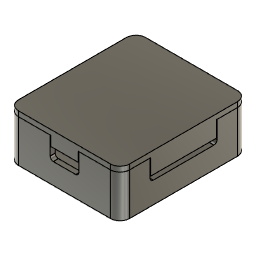
usbwledc-case (Autodesk Fusion 360 design; units mm, degrees)
Autodesk Fusion 360 part; units mm, degrees
sketch "Skizze1" plane through (0, 0, 0) normal (0, 0, 1) x (1, 0, 0)
  line L0 (0, 0) -> (34.8, 0)
  line L1 (34.8, 0) -> (34.8, 39.8)
  line L2 (34.8, 39.8) -> (0, 39.8)
  line L3 (0, 39.8) -> (0, 0)
  line L4 (33.2, 1.6) -> (1.6, 1.6)
  line L5 (1.6, 1.6) -> (1.6, 38.2)
  line L6 (1.6, 38.2) -> (33.2, 38.2)
  line L7 (33.2, 38.2) -> (33.2, 1.6)
  line L8 (33.2, 1.6) -> (1.6, 38.2) construction
  line L9 (1.6, 1.6) -> (33.2, 38.2) construction
  line L10 (33.2, 1.6) -> (29.4, 1.6) construction
  line L11 (29.4, 1.6) -> (29.4, 5.4) construction
  line L12 (1.6, 1.6) -> (5.4, 1.6) construction
  line L13 (5.4, 1.6) -> (5.4, 5.4) construction
  circle A0 centre (29.4, 5.4) radius 1.4
  circle A1 centre (5.4, 5.4) radius 1.4
  line L14 (5.4, 1.6) -> (7.9, 1.6) construction
  line L15 (7.9, 1.6) -> (7.9, 5.4)
  arc A2 (7.9, 5.4) -> (5.4, 7.9) centre (5.4, 5.4) ccw
  line L16 (5.4, 7.9) -> (1.6, 7.9)
  line L17 (29.4, 1.6) -> (26.9, 1.6) construction
  line L18 (33.2, 38.2) -> (29.4, 38.2) construction
  line L19 (1.6, 38.2) -> (5.4, 38.2) construction
  line L20 (5.4, 38.2) -> (5.4, 34.4) construction
  line L21 (29.4, 38.2) -> (29.4, 34.4) construction
  circle A3 centre (29.4, 34.4) radius 1.4
  circle A4 centre (5.4, 34.4) radius 1.4
  line L22 (29.4, 38.2) -> (26.9, 38.2) construction
  line L23 (5.4, 38.2) -> (7.9, 38.2) construction
  line L24 (26.9, 38.2) -> (26.9, 34.4)
  line L25 (7.9, 38.2) -> (7.9, 34.4)
  arc A5 (5.4, 31.9) -> (7.9, 34.4) centre (5.4, 34.4) ccw
  arc A6 (26.9, 34.4) -> (29.4, 31.9) centre (29.4, 34.4) ccw
  line L26 (5.4, 31.9) -> (1.6, 31.9)
  line L27 (29.4, 31.9) -> (33.2, 31.9)
  line L28 (26.9, 1.6) -> (26.9, 5.4)
  arc A7 (29.4, 7.9) -> (26.9, 5.4) centre (29.4, 5.4) ccw
  line L29 (29.4, 7.9) -> (33.2, 7.9)
  point P0 (17.4, 19.9)
  dimension "d15" = 34.8
  dimension "d16" = 39.8
  dimension "d17" = 31.6
  dimension "d18" = 36.6
  dimension "d19" = 3.8
  dimension "d20" = 3.8
  dimension "d21" = 3.8
  dimension "d22" = 3.8
  dimension "d23" = 2.8
  dimension "d24" = 2.8
  dimension "d27" = 2.5
  dimension "d28" = 3.8
  dimension "d29" = 2.5
  dimension "d30" = 3.8
  dimension "d31" = 3.8
  dimension "d32" = 3.8
  dimension "d33" = 3.8
  dimension "d34" = 2.8
  dimension "d35" = 2.8
  dimension "d36" = 2.5
  dimension "d37" = 2.5
  dimension "d38" = 3.8
  dimension "d39" = 3.8
  dimension "d40" = 3.8
  constraint horizontal L0
  constraint vertical L1
  constraint horizontal L2
  constraint vertical L3
  constraint coincident L0.start L3.end
  constraint horizontal L4
  constraint perpendicular L4 L5
  constraint parallel L4 L6
  constraint parallel L5 L7
  constraint coincident L8 P0
  constraint coincident L9 P0
  constraint perpendicular L7 L10
  constraint perpendicular L4 L11
  constraint perpendicular L5 L12
  constraint perpendicular L4 L13
  constraint coincident L11.end A0.centre
  constraint coincident L13.end A1.centre
  constraint perpendicular L13 L14
  constraint perpendicular L14 L15
  constraint coincident L5 L16.end
  constraint tangent A2 L16
  constraint perpendicular L5 L16
  constraint perpendicular L11 L17
  constraint perpendicular L7 L18
  constraint perpendicular L5 L19
  constraint perpendicular L19 L20
  constraint perpendicular L6 L21
  constraint coincident L21.end A3.centre
  constraint coincident L20.end A4.centre
  constraint perpendicular L21 L22
  constraint perpendicular L21 L23
  constraint perpendicular L22 L24
  constraint perpendicular L23 L25
  constraint coincident L5 L26.end
  constraint tangent A5 L26
  constraint perpendicular L5 L26
  constraint coincident L7 L27.end
  constraint tangent A6 L27
  constraint perpendicular L7 L27
  constraint perpendicular L17 L28
  constraint coincident L7 L29.end
  constraint tangent A7 L29
  constraint perpendicular L7 L29
  measures "d15" distance of L0.start L0.end
  measures "d16" distance of L0.start L2.end
  measures "d17" distance of L5.end L6.end
  measures "d18" distance of L4.end L5.end
  measures "d19" distance of L4.start L10.end
  measures "d20" distance of L10.end L11.end
  measures "d21" distance of L4.end L12.end
  measures "d22" distance of L12.end L13.end
  measures "d23" diameter of A0
  measures "d24" diameter of A1
  measures "d27" distance of L12.end L14.end
  measures "d28" distance of L14.end L15.end
  measures "d29" distance of L10.end L17.end
  measures "d30" distance of L6.end L18.end
  measures "d31" distance of L5.end L19.end
  measures "d32" distance of L19.end L20.end
  measures "d33" distance of L18.end L21.end
  measures "d34" diameter of A3
  measures "d35" diameter of A4
  measures "d36" distance of L18.end L22.end
  measures "d37" distance of L19.end L23.end
  measures "d38" distance of L22.end L24.end
  measures "d39" distance of L23.end L25.end
  measures "d40" distance of L17.end L28.end
extrude "Extrusion1" add sketch "Skizze1" along normal blind 1.6 contours L4 L5 L6 L7 L15 A2 L16 L24 L25 A5 A6 L26 L27 L28 A7 L29 makes body 1
extrude "Extrusion2" add sketch "Skizze1" along normal blind 5.1 contours L4 L7 L28 A7 L29 | L4 L5 L15 A2 L16 | L6 L7 L24 A6 L27 | L5 L6 L25 A5 L26 bodies 1
extrude "Extrusion3" add sketch "Skizze1" along normal blind 13.2 contours L0 L1 L2 L3 bodies 1
extrude "Extrusion4" add sketch "Skizze1" along normal blind 6.7 contours A0 | A1 | A3 | A4 bodies 1
sketch "Skizze2" plane through (0, 0, 1.6) normal (0, 0, 1) x (-1, 0, 0)
  line L0 (-26.9, -1.6) -> (-26.9, -5.4)
  arc A0 (-29.4, -7.9) -> (-26.9, -5.4) centre (-29.4, -5.4) ccw
  line L1 (-29.4, -7.9) -> (-33.2, -7.9)
  line L2 (-33.2, -7.9) -> (-33.2, -31.9)
  line L3 (-33.2, -31.9) -> (-29.4, -31.9)
  arc A1 (-26.9, -34.4) -> (-29.4, -31.9) centre (-29.4, -34.4) ccw
  line L4 (-26.9, -34.4) -> (-26.9, -38.2)
  line L5 (-26.9, -38.2) -> (-7.9, -38.2)
  line L6 (-7.9, -38.2) -> (-7.9, -34.4)
  arc A2 (-5.4, -31.9) -> (-7.9, -34.4) centre (-5.4, -34.4) ccw
  line L7 (-5.4, -31.9) -> (-1.6, -31.9)
  line L8 (-1.6, -31.9) -> (-1.6, -7.9)
  line L9 (-1.6, -7.9) -> (-5.4, -7.9)
  arc A3 (-7.9, -5.4) -> (-5.4, -7.9) centre (-5.4, -5.4) ccw
  line L10 (-7.9, -5.4) -> (-7.9, -1.6)
  line L11 (-7.9, -1.6) -> (-26.9, -1.6)
  line L12 (-33.2, -7.9) -> (-32.6, -7.9)
  line L13 (-32.6, -7.9) -> (-32.6, -31.9)
  line L14 (-32.6, -31.9) -> (-33.2, -31.9)
  line L15 (-33.2, -31.9) -> (-33.2, -7.9)
  dimension "d49" = 0.6
  constraint coincident L1.end L2.start
  constraint coincident L1 L12.end
  constraint coincident L3 L13.end
  constraint perpendicular L3 L13
  constraint coincident L2.end L3.start
  measures "d49" distance of L1.end L12.end
extrude "Extrusion5" add sketch "Skizze2" along normal blind 5.1 contours L1 L2 L3 L12 L13 L14 L15 bodies 1
sketch "Skizze3" plane through (0, 0, 0) normal (0, -1, 0) x (1, 0, 0)
  line L0 (0, 0) -> (34.8, 0)
  line L1 (34.8, 0) -> (34.8, 13.2)
  line L2 (34.8, 13.2) -> (0, 13.2)
  line L3 (0, 13.2) -> (0, 0)
  line L4 (17.4, 0) -> (17.4, 6.5) construction
  line L5 (17.4, 6.5) -> (21.9, 6.5)
  line L6 (17.4, 6.5) -> (12.9, 6.5)
  line L7 (12.9, 6.5) -> (12.9, 13.2)
  line L8 (21.9, 6.5) -> (21.9, 13.2)
  line L9 (21.9, 13.2) -> (12.9, 13.2)
  dimension "d52" = 6.5
  dimension "d55" = 4.5
  dimension "d56" = 4.5
  constraint midpoint L0 L4.start
  constraint perpendicular L0 L4
  constraint perpendicular L4 L5
  constraint perpendicular L4 L6
  constraint coincident L2 L7.end
  constraint perpendicular L2 L7
  constraint coincident L2 L8.end
  constraint perpendicular L2 L8
  measures "d52" distance of L4.start L4.end
  measures "d55" distance of L4.end L5.end
  measures "d56" distance of L4.end L6.end
extrude "Extrusion6" cut sketch "Skizze3" against normal blind 1.6 contours L2 L5 L6 L7 L8 L9 bodies 1
sketch "Skizze4" plane through (34.8, 0, 0) normal (1, 0, 0) x (0, 1, 0)
  line L0 (0, 0) -> (39.8, 0)
  line L1 (39.8, 0) -> (39.8, 13.2)
  line L2 (39.8, 13.2) -> (0, 13.2)
  line L3 (0, 13.2) -> (0, 0)
  line L4 (19.9, 0) -> (19.9, 6.7) construction
  line L5 (19.9, 6.7) -> (30.4, 6.7)
  line L6 (19.9, 6.7) -> (9.4, 6.7)
  line L7 (9.4, 6.7) -> (9.4, 13.2)
  line L8 (30.4, 6.7) -> (30.4, 13.2)
  line L9 (30.4, 13.2) -> (9.4, 13.2)
  dimension "d59" = 6.7
  dimension "d60" = 10.5
  dimension "d61" = 10.5
  constraint midpoint L0 L4.start
  constraint perpendicular L0 L4
  constraint perpendicular L1 L5
  constraint perpendicular L4 L6
  constraint coincident L2 L7.end
  constraint perpendicular L2 L7
  constraint coincident L2 L8.end
  constraint perpendicular L2 L8
  measures "d59" distance of L4.start L4.end
  measures "d60" distance of L4.end L5.end
  measures "d61" distance of L4.end L6.end
extrude "Extrusion7" cut sketch "Skizze4" against normal blind 1.6 contours L2 L5 L6 L7 L8 L9 bodies 1
ref_plane "Arbeitsebene1" through (0, 0, 13.2) normal (0, 0, 1) x (1, 0, 0)
ref_plane "Arbeitsebene2" through (0, 19.9, 0) normal (0, 1, 0) x (0, 0, 1)
sketch "Skizze6" plane through (0, 0, 13.2) normal (0, 0, 1) x (1, 0, 0)
  line L0 (2, 2) -> (2, 37.8)
  line L1 (5.4, 2) -> (5.4, 5.4) construction
  line L2 (32.8, 37.8) -> (32.8, 2)
  line L3 (29.4, 2) -> (26.9, 2) construction
  line L4 (29.4, 7.9) -> (32.8, 7.9)
  line L5 (32.8, 37.8) -> (29.4, 37.8) construction
  line L6 (5.4, 2) -> (7.9, 2) construction
  line L7 (32.8, 2) -> (29.4, 2) construction
  line L8 (34.8, 0) -> (34.8, 39.8)
  line L9 (2, 37.8) -> (5.4, 37.8) construction
  line L10 (5.4, 37.8) -> (7.9, 37.8) construction
  arc A0 (29.4, 7.9) -> (26.9, 5.4) centre (29.4, 5.4) ccw
  line L11 (29.4, 2) -> (29.4, 5.4) construction
  line L12 (0, 39.8) -> (0, 0)
  line L13 (26.9, 2) -> (26.9, 5.4)
  line L14 (2, 2) -> (5.4, 2) construction
  line L15 (2, 2) -> (32.8, 37.8) construction
  line L16 (2, 37.8) -> (32.8, 37.8)
  line L17 (34.8, 39.8) -> (0, 39.8)
  line L18 (0, 0) -> (34.8, 0)
  line L19 (32.8, 2) -> (2, 37.8) construction
  line L20 (32.8, 2) -> (2, 2)
  line L21 (29.4, 37.8) -> (26.9, 37.8) construction
  line L22 (7.9, 2) -> (7.9, 5.4)
  arc A1 (7.9, 5.4) -> (5.4, 7.9) centre (5.4, 5.4) ccw
  line L23 (5.4, 5.4) -> (7.9, 5.4) construction
  line L24 (5.4, 5.4) -> (5.4, 7.9) construction
  line L25 (5.4, 7.9) -> (2, 7.9)
  line L26 (7.9, 37.8) -> (7.9, 34.4)
  line L27 (26.9, 37.8) -> (26.9, 34.4)
  line L28 (29.4, 37.8) -> (29.4, 34.4) construction
  line L29 (5.4, 37.8) -> (5.4, 34.4) construction
  arc A2 (5.4, 31.9) -> (7.9, 34.4) centre (5.4, 34.4) ccw
  line L30 (5.4, 34.4) -> (5.4, 31.9) construction
  line L31 (5.4, 34.4) -> (7.9, 34.4) construction
  arc A3 (26.9, 34.4) -> (29.4, 31.9) centre (29.4, 34.4) ccw
  line L32 (29.4, 34.4) -> (26.9, 34.4) construction
  line L33 (29.4, 34.4) -> (29.4, 31.9) construction
  line L34 (5.4, 31.9) -> (2, 31.9)
  line L35 (29.4, 31.9) -> (32.8, 31.9)
  point P0 (17.4, 19.9)
  dimension "d89" = 34.8
  dimension "d90" = 39.8
  dimension "d91" = 30.8
  dimension "d92" = 35.8
  dimension "d93" = 3.4
  dimension "d94" = 3.4
  dimension "d95" = 3.4
  dimension "d96" = 3.4
  dimension "d99" = 2.5
  dimension "d101" = 2.5
  dimension "d102" = 3.4
  dimension "d103" = 3.4
  dimension "d108" = 2.5
  dimension "d109" = 2.5
  dimension "d112" = 3.4
  dimension "d118" = 3.4
  dimension "d119" = 90
  dimension "d120" = 3.4
  dimension "d121" = 3.4
  dimension "d122" = 3.4
  dimension "d123" = 3.4
  dimension "d124" = 90
  dimension "d125" = 90
  constraint horizontal L18
  constraint vertical L8
  constraint horizontal L17
  constraint vertical L12
  constraint coincident L12.end L18.start
  constraint horizontal L20
  constraint perpendicular L0 L20
  constraint parallel L16 L20
  constraint parallel L0 L2
  constraint coincident P0 L19
  constraint coincident P0 L15
  constraint perpendicular L2 L7
  constraint perpendicular L11 L20
  constraint perpendicular L0 L14
  constraint perpendicular L1 L20
  constraint perpendicular L1 L6
  constraint perpendicular L3 L11
  constraint perpendicular L2 L5
  constraint perpendicular L0 L9
  constraint perpendicular L3 L13
  constraint coincident L4.end L2
  constraint tangent L4 A0
  constraint perpendicular L2 L4
  constraint perpendicular L20 L22
  constraint coincident L0 L25.end
  constraint tangent A1 L25
  constraint perpendicular L10 L26
  constraint perpendicular L21 L27
  constraint perpendicular L5 L28
  constraint perpendicular L10 L29
  constraint coincident L29.end A2.centre
  constraint coincident L28.end A3.centre
  constraint coincident L0 L34.end
  constraint tangent A2 L34
  constraint perpendicular L0 L34
  constraint coincident L2 L35.end
  constraint tangent A3 L35
  constraint perpendicular L2 L35
  measures "d89" distance of L8.start L12.end
  measures "d90" distance of L12.end L12.start
  measures "d91" distance of L2.start L0.end
  measures "d92" distance of L0.start L0.end
  measures "d93" distance of L2.end L3.start
  measures "d94" distance of L3.start A0.centre
  measures "d95" distance of L0.start L1.start
  measures "d96" distance of L1.start L1.end
  measures "d99" distance of L1.start L6.end
  measures "d101" distance of L3.end L3.start
  measures "d102" distance of L2.start L5.end
  measures "d103" distance of L0.end L9.end
  measures "d108" distance of L21.end L5.end
  measures "d109" distance of L10.end L9.end
  measures "d112" distance of L3.end A0.end
  measures "d118" distance of L6.end L22.end
  measures "d119" angle of L23 L24
  measures "d120" distance of L10.end L26.end
  measures "d121" distance of L21.end L27.end
  measures "d122" distance of L5.end L28.end
  measures "d123" distance of L9.end L29.end
  measures "d124" angle of L30 L31
  measures "d125" angle of L32 L33
extrude "Extrusion8" add sketch "Skizze6" along normal blind 1.6 separate body contours L0 L20 L22 A1 L25 | L0 L2 L4 A0 L13 L16 L20 L22 A1 L25 L26 L27 A2 A3 L34 L35 | L0 L16 L26 A2 L34 | L2 L4 A0 L13 L20 | L2 L16 L27 A3 L35 | L8 L12 L17 L18 makes body 2
extrude "Extrusion9" add sketch "Skizze6" against normal blind 6.4 contours L0 L20 L22 A1 L25 | L0 L16 L26 A2 L34 | L2 L4 A0 L13 L20 | L2 L16 L27 A3 L35 bodies 2
ref_plane "Arbeitsebene3" through (0, 0, 6.7) normal (0, 0, 1) x (1, 0, 0)
sketch "Skizze7" plane through (0, 0, 13.2) normal (0, 0, -1) x (1, 0, 0)
  line L0 (32.8, -37.8) -> (26.9, -37.8)
  line L1 (26.9, -37.8) -> (26.9, -34.4)
  arc A0 (29.4, -31.9) -> (26.9, -34.4) centre (29.4, -34.4) ccw
  line L2 (29.4, -31.9) -> (32.8, -31.9)
  line L3 (32.8, -31.9) -> (32.8, -37.8)
  line L4 (2, -2) -> (7.9, -2)
  line L5 (7.9, -2) -> (7.9, -5.4)
  arc A1 (5.4, -7.9) -> (7.9, -5.4) centre (5.4, -5.4) ccw
  line L6 (5.4, -7.9) -> (2, -7.9)
  line L7 (2, -7.9) -> (2, -2)
  line L8 (26.9, -5.4) -> (26.9, -2)
  line L9 (26.9, -2) -> (32.8, -2)
  line L10 (32.8, -2) -> (32.8, -7.9)
  line L11 (32.8, -7.9) -> (29.4, -7.9)
  arc A2 (26.9, -5.4) -> (29.4, -7.9) centre (29.4, -5.4) ccw
  line L12 (7.9, -34.4) -> (7.9, -37.8)
  line L13 (7.9, -37.8) -> (2, -37.8)
  line L14 (2, -37.8) -> (2, -31.9)
  line L15 (2, -31.9) -> (5.4, -31.9)
  arc A3 (7.9, -34.4) -> (5.4, -31.9) centre (5.4, -34.4) ccw
  line L16 (34.8, 0) -> (0, 0)
  line L17 (0, 0) -> (0, -39.8)
  line L18 (0, -39.8) -> (34.8, -39.8)
  line L19 (34.8, -39.8) -> (34.8, 0)
  line L20 (17.4, 0) -> (21.7, 0)
  line L21 (21.7, 0) -> (21.7, -1.6)
  line L22 (21.7, -1.6) -> (13.1, -1.6)
  line L23 (13.1, -1.6) -> (13.1, 0)
  line L24 (13.1, 0) -> (17.4, 0)
  dimension "d127" = 4.3
  dimension "d128" = 1.6
  dimension "d129" = 8.6
  constraint midpoint L16 L20.start
  constraint coincident L16 L20.end
  constraint perpendicular L20 L21
  constraint perpendicular L21 L22
  constraint coincident L16 L23.end
  constraint perpendicular L16 L23
  measures "d127" distance of L20.start L20.end
  measures "d128" distance of L20.end L21.end
  measures "d129" distance of L21.end L22.end
extrude "Extrusion10" add sketch "Skizze7" along normal blind 3 contours L16 L20 L21 L22 L23 L24 bodies 2
sketch "Skizze8" plane through (0, 0, 13.2) normal (0, 0, -1) x (1, 0, 0)
  line L0 (21.7, 0) -> (21.7, -1.6)
  line L1 (21.7, -1.6) -> (13.1, -1.6)
  line L2 (13.1, -1.6) -> (13.1, 0)
  line L3 (13.1, 0) -> (0, 0)
  line L4 (0, 0) -> (0, -39.8)
  line L5 (0, -39.8) -> (34.8, -39.8)
  line L6 (34.8, -39.8) -> (34.8, 0)
  line L7 (34.8, 0) -> (21.7, 0)
  line L8 (7.9, -34.4) -> (7.9, -37.8)
  line L9 (7.9, -37.8) -> (2, -37.8)
  line L10 (2, -37.8) -> (2, -31.9)
  line L11 (2, -31.9) -> (5.4, -31.9)
  arc A0 (7.9, -34.4) -> (5.4, -31.9) centre (5.4, -34.4) ccw
  line L12 (26.9, -5.4) -> (26.9, -2)
  line L13 (26.9, -2) -> (32.8, -2)
  line L14 (32.8, -2) -> (32.8, -7.9)
  line L15 (32.8, -7.9) -> (29.4, -7.9)
  arc A1 (26.9, -5.4) -> (29.4, -7.9) centre (29.4, -5.4) ccw
  line L16 (2, -2) -> (7.9, -2)
  line L17 (7.9, -2) -> (7.9, -5.4)
  arc A2 (5.4, -7.9) -> (7.9, -5.4) centre (5.4, -5.4) ccw
  line L18 (5.4, -7.9) -> (2, -7.9)
  line L19 (2, -7.9) -> (2, -2)
  line L20 (32.8, -37.8) -> (26.9, -37.8)
  line L21 (26.9, -37.8) -> (26.9, -34.4)
  arc A3 (29.4, -31.9) -> (26.9, -34.4) centre (29.4, -34.4) ccw
  line L22 (29.4, -31.9) -> (32.8, -31.9)
  line L23 (32.8, -31.9) -> (32.8, -37.8)
  line L24 (34.8, -19.9) -> (34.8, -30.2)
  line L25 (34.8, -30.2) -> (32.6, -30.2)
  line L26 (32.6, -30.2) -> (32.6, -9.6)
  line L27 (32.6, -9.6) -> (34.8, -9.6)
  line L28 (34.8, -9.6) -> (34.8, -19.9)
  dimension "d132" = 10.3
  dimension "d133" = 2.2
  dimension "d134" = 20.6
  constraint midpoint L6 L24.start
  constraint parallel L6 L24
  constraint perpendicular L24 L25
  constraint perpendicular L25 L26
  constraint coincident L6 L27.end
  constraint perpendicular L6 L27
  measures "d132" distance of L24.start L24.end
  measures "d133" distance of L24.end L25.end
  measures "d134" distance of L25.end L26.end
extrude "Extrusion11" add sketch "Skizze8" along normal blind 5 contours L6 L24 L25 L26 L27 L28 bodies 2
sketch "Skizze9" plane through (32.8, 0, 0) normal (1, 0, 0) x (0, 1, 0)
  line L0 (7.9, 13.2) -> (2, 13.2)
  line L1 (2, 13.2) -> (2, 6.8)
  line L2 (2, 6.8) -> (7.9, 6.8)
  line L3 (7.9, 6.8) -> (7.9, 13.2)
  line L4 (2, 13.2) -> (7.9, 6.8) construction
  line L5 (2, 6.8) -> (7.9, 13.2) construction
  constraint coincident L0.end L1.start
  constraint coincident L2.end L3.start
  constraint coincident L1.end L2.start
  constraint coincident L0.start L3.end
sketch "Skizze10" plane through (32.8, 0, 0) normal (1, 0, 0) x (0, 1, 0)
  line L0 (37.8, 13.2) -> (31.9, 13.2)
  line L1 (31.9, 13.2) -> (31.9, 6.8)
  line L2 (31.9, 6.8) -> (37.8, 6.8)
  line L3 (37.8, 6.8) -> (37.8, 13.2)
  line L4 (31.9, 13.2) -> (37.8, 6.8) construction
  line L5 (31.9, 6.8) -> (37.8, 13.2) construction
  constraint coincident L0.end L1.start
  constraint coincident L2.end L3.start
  constraint coincident L1.end L2.start
  constraint coincident L0.start L3.end
sketch "Skizze11" plane through (2, 0, 0) normal (-1, 0, 0) x (0, -1, 0)
  line L0 (-31.9, 13.2) -> (-37.8, 13.2)
  line L1 (-37.8, 13.2) -> (-37.8, 6.8)
  line L2 (-37.8, 6.8) -> (-31.9, 6.8)
  line L3 (-31.9, 6.8) -> (-31.9, 13.2)
  line L4 (-37.8, 6.8) -> (-31.9, 13.2) construction
  line L5 (-37.8, 13.2) -> (-31.9, 6.8) construction
  constraint coincident L1.end L2.start
  constraint coincident L0.start L3.end
  constraint coincident L0.end L1.start
  constraint coincident L2.end L3.start
sketch "Skizze12" plane through (2, 0, 0) normal (-1, 0, 0) x (0, -1, 0)
  line L0 (-2, 13.2) -> (-7.9, 13.2)
  line L1 (-7.9, 13.2) -> (-7.9, 6.8)
  line L2 (-7.9, 6.8) -> (-2, 6.8)
  line L3 (-2, 6.8) -> (-2, 13.2)
  line L4 (-7.9, 13.2) -> (-2, 6.8) construction
  line L5 (-7.9, 6.8) -> (-2, 13.2) construction
  constraint coincident L0.end L1.start
  constraint coincident L2.end L3.start
  constraint coincident L1.end L2.start
  constraint coincident L0.start L3.end
sphere "Grundkörper Kugel1" add diameter 2.4 placed x (0, -1, 0) y (0, 0, 1) z (-1, 0, 0) at (2, 4.95, 10) bodies 2
sphere "Grundkörper Kugel2" add diameter 2.4 placed x (0, -1, 0) y (0, 0, 1) z (-1, 0, 0) at (2, 34.85, 10) bodies 2
sphere "Grundkörper Kugel3" add diameter 2.4 placed x (0, 1, 0) y (0, 0, 1) z (1, 0, 0) at (32.8, 4.95, 10) bodies 2
sphere "Grundkörper Kugel4" add diameter 2.4 placed x (0, 1, 0) y (0, 0, 1) z (1, 0, 0) at (32.8, 34.85, 10) bodies 2
sphere "Grundkörper Kugel5" cut diameter 2.5 placed x (0, -1, 0) y (0, 0, 1) z (-1, 0, 0) at (2, 4.95, 10) bodies 1
sphere "Grundkörper Kugel6" cut diameter 2.5 placed x (0, -1, 0) y (0, 0, 1) z (-1, 0, 0) at (2, 34.85, 10) bodies 1
sphere "Grundkörper Kugel7" cut diameter 2.5 placed x (0, 1, 0) y (0, 0, 1) z (1, 0, 0) at (32.8, 4.95, 10) bodies 1
sphere "Grundkörper Kugel8" cut diameter 2.5 placed x (0, 1, 0) y (0, 0, 1) z (1, 0, 0) at (32.8, 34.85, 10) bodies 1
fillet "Abrundung1" radius 1.5 8 edges at (33.2, 1.6, 9.15) (33.2, 38.2, 9.15) (1.6, 38.2, 9.15) (1.6, 1.6, 9.15) (32.8, 37.8, 10) (32.8, 2, 10) (2, 37.8, 10) (2, 2, 10) on bodies 1 2
fillet "Abrundung2" radius 3 8 edges at (0, 39.8, 6.6) (34.8, 39.8, 6.6) (0, 0, 6.6) (34.8, 0, 6.6) (0, 39.8, 14) (34.8, 39.8, 14) (0, 0, 14) (34.8, 0, 14) on bodies 1 2
fillet "Abrundung3" radius 2.5 1 edges at (32.6, 19.9, 13.2) on bodies 2
fillet "Abrundung4" radius 1 2 edges at (21.9, 0.8, 6.5) (12.9, 0.8, 6.5) on bodies 1
fillet "Abrundung5" radius 1 2 edges at (34, 30.4, 6.7) (34, 9.4, 6.7) on bodies 1
equation "platineBreite = 30 mm"
equation "platineLänge = 35 mm"
equation "platineAbstandUnten = 3.5 mm"
equation "platineAbstandOben = 6.5 mm"
equation "platineLochAbstand = 3 mm"
equation "platineLochDurchmesser = 3.2 mm"
equation "platineDicke = 1.6 mm"
equation "wandstärke = 1.6 mm"
equation "platineAbstandBreite = 0.8 mm"
equation "platineAbstandLänge = platineAbstandBreite"
equation "platinePadsLänge = 21 mm"
equation "platineKabelDicke = 1.5 mm"
equation "toleranz = 0.2 mm"
equation "d15 = platineBreite + ( ( wandstärke + platineAbstandBreite ) * 2 )"
equation "d16 = platineLänge + ( ( platineAbstandLänge + wandstärke ) * 2 )"
equation "d17 = platineBreite + ( platineAbstandBreite * 2 )"
equation "d18 = platineLänge + ( platineAbstandLänge * 2 )"
equation "d19 = platineLochAbstand + platineAbstandBreite"
equation "d20 = platineAbstandLänge + platineLochAbstand"
equation "d21 = platineLochAbstand + platineAbstandBreite"
equation "d22 = platineLochAbstand + platineAbstandLänge"
equation "d23 = platineLochDurchmesser - ( toleranz * 2 )"
equation "d24 = platineLochDurchmesser - ( toleranz * 2 )"
equation "platineLochRing = 5 mm"
equation "d27 = platineLochRing / 2"
equation "d28 = platineLochAbstand + platineAbstandLänge"
equation "d29 = platineLochRing / 2"
equation "d30 = platineLochAbstand + platineAbstandBreite"
equation "d31 = platineLochAbstand + platineAbstandBreite"
equation "d32 = platineLochAbstand + platineAbstandLänge"
equation "d33 = platineLochAbstand + platineAbstandLänge"
equation "d34 = platineLochDurchmesser - ( 2 * toleranz )"
equation "d35 = platineLochDurchmesser - ( 2 * toleranz )"
equation "d36 = platineLochRing / 2"
equation "d37 = platineLochRing / 2"
equation "d38 = platineLochAbstand + platineAbstandLänge"
equation "d39 = platineLochAbstand + platineAbstandLänge"
equation "d40 = platineAbstandLänge + platineLochAbstand"
equation "d41 = wandstärke"
equation "d43 = wandstärke + platineAbstandUnten"
equation "d45 = wandstärke + platineAbstandUnten + platineDicke + platineAbstandOben"
equation "d47 = wandstärke + platineAbstandUnten + platineDicke"
equation "d49 = platineAbstandBreite - toleranz"
equation "d50 = platineAbstandUnten + platineDicke"
equation "d52 = wandstärke + platineAbstandUnten + platineDicke - toleranz"
equation "usbbreite = 9 mm"
equation "usbhöhe = 3.3 mm"
equation "d55 = usbbreite / 2"
equation "d56 = usbbreite / 2"
equation "d57 = -wandstärke"
equation "d59 = wandstärke + platineAbstandUnten + platineDicke"
equation "d60 = platinePadsLänge / 2"
equation "d61 = platinePadsLänge / 2"
equation "d62 = -wandstärke"
equation "d88 = wandstärke + platineAbstandUnten + platineDicke + platineAbstandOben"
equation "d89 = platineBreite + ( ( wandstärke + platineAbstandBreite ) * 2 )"
equation "d90 = platineLänge + ( ( platineAbstandLänge + wandstärke ) * 2 )"
equation "d91 = platineBreite + ( platineAbstandBreite * 2 ) - ( 4 * toleranz )"
equation "d92 = platineLänge + ( platineAbstandLänge * 2 ) - ( 4 * toleranz )"
equation "d93 = platineLochAbstand + platineAbstandBreite - ( 2 * toleranz )"
equation "d94 = platineAbstandLänge + platineLochAbstand - ( 2 * toleranz )"
equation "d95 = platineLochAbstand + platineAbstandBreite - ( 2 * toleranz )"
equation "d96 = platineLochAbstand + platineAbstandLänge - ( 2 * toleranz )"
equation "d99 = platineLochRing / 2"
equation "d101 = platineLochRing / 2"
equation "d102 = platineLochAbstand + platineAbstandBreite - ( 2 * toleranz )"
equation "d103 = platineLochAbstand + platineAbstandBreite - ( 2 * toleranz )"
equation "d108 = platineLochRing / 2"
equation "d109 = platineLochRing / 2"
equation "d112 = platineAbstandLänge + platineLochAbstand - ( 2 * toleranz )"
equation "d113 = wandstärke"
equation "d115 = -platineAbstandOben + ( toleranz / 2 )"
equation "d117 = wandstärke + ( platineLänge / 2 ) + platineAbstandLänge"
equation "d118 = platineLochAbstand + platineAbstandLänge - ( 2 * toleranz )"
equation "d120 = platineLochAbstand + platineAbstandLänge - ( 2 * toleranz )"
equation "d121 = platineLochAbstand + platineAbstandLänge - ( 2 * toleranz )"
equation "d122 = platineLochAbstand + platineAbstandLänge - ( 2 * toleranz )"
equation "d123 = platineLochAbstand + platineAbstandLänge - ( 2 * toleranz )"
equation "d126 = wandstärke + platineAbstandUnten + platineDicke"
equation "d127 = ( usbbreite / 2 ) - toleranz"
equation "d128 = wandstärke"
equation "d129 = usbbreite - ( 2 * toleranz )"
equation "d130 = platineAbstandOben - usbhöhe - toleranz"
equation "d132 = ( platinePadsLänge / 2 ) - toleranz"
equation "d133 = wandstärke + platineAbstandBreite - toleranz"
equation "d134 = platinePadsLänge - ( 2 * toleranz )"
equation "d135 = platineAbstandOben - platineKabelDicke"
equation "d141 = 2.40 mm + ( toleranz / 2 )"
equation "d142 = 2.40 mm + ( toleranz / 2 )"
equation "d143 = 2.40 mm + ( toleranz / 2 )"
equation "d144 = 2.40 mm + ( toleranz / 2 )"
named bodies: "Basis", "Deckel"
